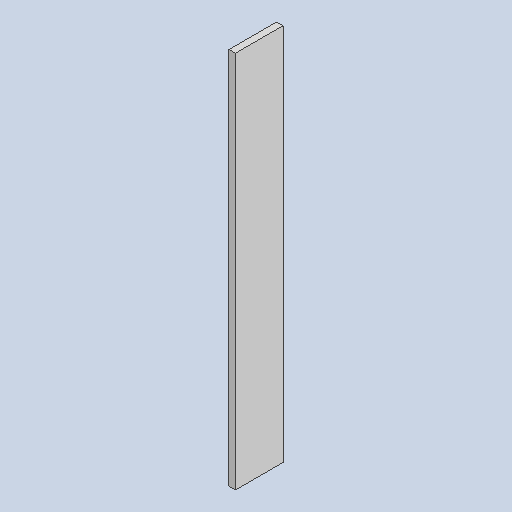
# Autodesk Inventor part: ДМФ 01 58 Фиксатор расстояния кассет
Saved by Autodesk Inventor 2024.2 (Build 282272000, 272)
## iProperties
Created: 2024-05-05
Part Number: ДМФ 01 58 Фиксатор расстояния кассет
Material: Generic
Document SubType Name: Modeling
Designer: pokla
Density: 1 g/cm^3
Appearance: Default
Author: pokla
Autodesk Inventor part; units mm, degrees
ref_plane "YZ Plane" through (0, 0, 0) normal (1, 0, 0) x (0, 1, 0)
ref_plane "XZ Plane" through (0, 0, 0) normal (0, 1, 0) x (-1, 0, 0)
ref_plane "XY Plane" through (0, 0, 0) normal (0, 0, 1) x (1, 0, 0)
sketch "Sketch1" plane through (0, 0, 0) normal (0, 0, 1) x (1, 0, 0)
  line L0 (0, 273.8452) -> (193.6378, 193.6378) construction
  line L1 (193.6378, 193.6378) -> (273.8452, 0) construction
  line L2 (273.8452, 0) -> (193.6378, -193.6378) construction
  line L3 (193.6378, -193.6378) -> (0, -273.8452) construction
  line L4 (0, -273.8452) -> (-193.6378, -193.6378) construction
  line L5 (-193.6378, -193.6378) -> (-273.8452, 0) construction
  line L6 (-273.8452, 0) -> (-193.6378, 193.6378) construction
  line L7 (-193.6378, 193.6378) -> (0, 273.8452) construction
  line L8 (-193.6378, 193.6378) -> (0, 273.8452) construction
  line L9 (-459.9272, 770.6562) -> (-219.7185, 870.1539) construction
  line L10 (-96.8189, 233.7415) -> (-339.8229, 820.405) construction
  line L11 (-219.7185, 870.1539) -> (0, 870.1539) construction
  line L12 (0, 870.1539) -> (0, 273.8452) construction
  line L13 (-459.9272, 770.6562) -> (-615.2917, 615.2917) construction
  line L14 (-615.2917, 615.2917) -> (-193.6378, 193.6378) construction
  line L15 (-5, 865.1539) -> (-218.724, 865.1539) construction
  line L16 (-218.724, 865.1539) -> (-457.095, 766.4174) construction
  line L17 (-457.095, 766.4174) -> (-608.2206, 615.2917) construction
  line L18 (-608.2206, 615.2917) -> (-192.4647, 199.5357) construction
  line L19 (-192.4647, 199.5357) -> (-5, 277.1861) construction
  line L20 (-5, 277.1861) -> (-5, 865.1539)
  line L21 (-5, 865.1539) -> (-5, 277.1861) construction
  line L22 (5, 865.1539) -> (5, 277.1861)
  line L23 (-5, 277.1861) -> (5, 277.1861)
  line L24 (-5, 865.1539) -> (5, 865.1539)
  point P0 (0, 0)
  point P1 (0, 0)
  point P2 (0, 0)
  dimension "d0" = 506
  dimension "d1" = 260
  dimension "d2" = 635
  dimension "d6" = 5
  constraints: 50 end point, 3 horizontal, 2 coincident, 2 midpoint, 2 parallel, 2 vertical, 1 collinear, 1 horizontal alignment, 1 perpendicular, 1 symmetric about line, 1 vertical alignment, 23 other
  measures "d0" distance between parallel lines of L5 L1
  measures "d1" distance of L9.start L11.start
  measures "d2" distance of L10.end L10.start
  measures "d6" distance between parallel lines of L11 L15
extrude "Extrusion1" add sketch "Sketch1" along normal mid plane 74
equation "\"d0\" = Барабан_габарит_по_кассетам"
equation "\"d1\" = Кассета_длина_грани"
equation "\"d2\" = Кассета_высота"
equation "\"Барабан_габарит_по_кассетам\" = 506"
equation "\"Кассета_длина_грани\" = 260"
equation "\"Кассета_высота\" = 635"
body "Solid1"
